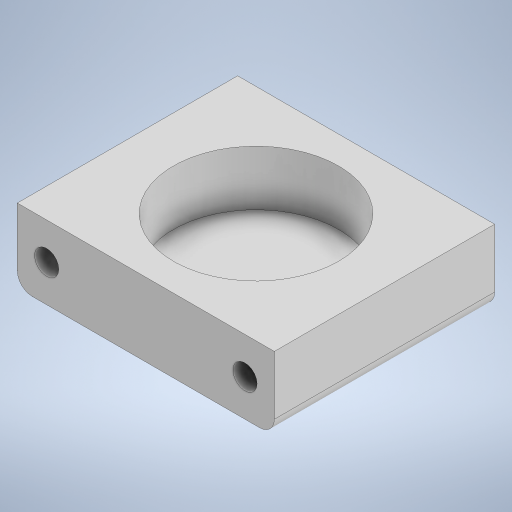
# Autodesk Inventor part: servo_pressfit_plate
Saved by Autodesk Inventor 2023 (Build 270158000, 158)
## iProperties
Created: 2023-02-02
Part Number: servo_pressfit_plate
Material: Generic
Document SubType Name: Modeling
Designer: Hunter
Density: 1 g/cm^3
Appearance: Default
Author: Hunter
Autodesk Inventor part; units mm, degrees
ref_plane "YZ Plane" through (0, 0, 0) normal (1, 0, 0) x (0, 1, 0)
ref_plane "XZ Plane" through (0, 0, 0) normal (0, 1, 0) x (-1, 0, 0)
ref_plane "XY Plane" through (0, 0, 0) normal (0, 0, 1) x (1, 0, 0)
sketch "Sketch1" plane through (0, 0, 0) normal (0, 0, 1) x (1, 0, 0)
  line L0 (-35, 0) -> (0, 0)
  line L1 (0, 0) -> (0, 10)
  line L2 (0, 10) -> (-35, 10)
  line L3 (-35, 10) -> (-35, 0)
  dimension "d0" = 35
  dimension "d1" = 10
  constraints: 8 end point, 2 parallel, 1 coincident, 1 horizontal, 1 perpendicular
  measures "d0" distance of L0.start L0.end
  measures "d1" distance of L2.end L0.start
extrude "Extrusion1" add sketch "Sketch1" along normal blind 30
sketch "Sketch2" plane through (-35, 10, 0) normal (0, 1, 0) x (1, 0, 0)
  line L0 (35, -30) -> (0, -30) construction
  line L1 (17.5, -30) -> (17.5, 0) construction
  line L2 (0, 0) -> (35, 0) construction
  circle A0 centre (17.5, -15) radius 11.25
  point P0 (30, -30)
  point P1 (5, -30)
  point P2 (5, 0)
  point P3 (30, 0)
  dimension "d5" = 22.5
  constraints: 3 midpoint, 2 end point, 1 centre point
  measures "d5" diameter of A0
extrude "Extrusion2" cut sketch "Sketch2" against normal blind 7.5
sketch "Sketch3" plane through (0, 0, 0) normal (0, 0, -1) x (-1, 0, 0)
  line L0 (0, 10) -> (35, 10) construction
  line L1 (17.5, 10) -> (17.5, 0) construction
  line L2 (30, 0) -> (5, 0) construction
  circle A0 centre (4, 5) radius 1.65
  circle A1 centre (31, 5) radius 1.65
  line L3 (0, 0) -> (0, 10) projected
  line L4 (35, 10) -> (35, 0) projected
  point P0 (5, 10)
  point P1 (30, 10)
  point P2 (17.5, 5)
  point P3 (0, 5)
  point P4 (35, 5)
  dimension "d8" = 3.3
  dimension "d9" = 4
  dimension "d10" = 4
  constraints: 3 midpoint, 2 centre point, 2 end point, 2 horizontal alignment, 1 equal radius
  measures "d8" diameter of A0
  measures "d9" distance from line of L3 A0.centre
  measures "d10" distance from line of L4 A1.centre
extrude "Extrusion3" cut sketch "Sketch3" against normal through all
fillet "Fillet2" radius 2 2 edges at (-35, 0, 15) (0, 0, 15)
body "Solid1"
